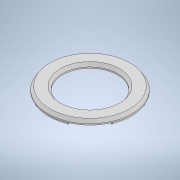
# Autodesk Inventor part: mirror_lock_v1
Saved by Autodesk Inventor 2020 (Build 240168000, 168)
## iProperties
Created: 2024-03-22
Part Number: mirror_lock_v1
Material: Типовые
Document SubType Name: Modeling
Designer: 4s
Density: 1 g/cm^3
Appearance: По умолчанию
Author: 4s
Autodesk Inventor part; units mm, degrees
ref_plane "YZ Plane" through (0, 0, 0) normal (1, 0, 0) x (0, 1, 0)
ref_plane "XZ Plane" through (0, 0, 0) normal (0, 1, 0) x (-1, 0, 0)
ref_plane "XY Plane" through (0, 0, 0) normal (0, 0, 1) x (1, 0, 0)
sketch "Эскиз1" plane through (0, 0, 0) normal (1, 0, 0) x (0, 1, 0)
  line L0 (0, 0) -> (13.9611, 0) construction
  line L1 (0, 26.35) -> (-10, 26.35) construction
  line L2 (-10, 26.35) -> (-10, -26.35) construction
  line L3 (-10, -26.35) -> (0, -26.35) construction
  line L4 (0, -26.35) -> (0, 26.35) construction
  line L5 (0, 0) -> (0, -22.0675) construction
  line L6 (2, 25) -> (0, 25) construction
  line L7 (0, 25) -> (0, -25) construction
  line L8 (0, -25) -> (2, -25) construction
  line L9 (2, -25) -> (2, 25) construction
  line L10 (5, -19) -> (5, -30.35)
  line L11 (-2, -11.433) -> (-2, -38.2242) construction
  line L12 (5, -19) -> (2, -19)
  line L13 (5, -30.35) -> (2, -30.35)
  line L14 (2, -30.35) -> (2, -19)
  dimension "d0" = 10
  dimension "d1" = 52.7
  dimension "d2" = 2
  dimension "d3" = 50
  dimension "d4" = 3
  dimension "d6" = 2
  dimension "d7" = 6
  dimension "d8" = 3
  dimension "d10" = 4
  constraints: 30 end point, 6 parallel, 4 horizontal, 3 perpendicular, 2 collinear, 2 vertical, 1 point on line, 2 other
  measures "d0" distance of L3.end L2.end
  measures "d1" distance of L3.end L1.start
  measures "d2" distance between parallel lines of L4 L9
  measures "d3" distance of L8.end L6.start
  measures "d4" distance between parallel lines of L9 L10
  measures "d6" distance between parallel lines of L4 L11
  measures "d7" distance between parallel lines of L8 L12
  measures "d8" distance of L10.end L13.end
  measures "d10" distance between parallel lines of L3 L13
revolve "Вращение1" add sketch "Эскиз1" angle 360 about axis through (0, 0, 0) along (0, 1, 0)
chamfer "Фаска1" distance 1.5 angle 55 1 edges at (0, 5, 19) measured on face at (0, 5, 19.5)
sketch "Эскиз2" plane through (0, 0, 0) normal (0, 0, 1) x (1, 0, 0)
  line L0 (-30.35, 5) -> (30.35, 5) construction
  line L1 (-30.35, 2) -> (30.35, 2) construction
  line L2 (-19, 2.8578) -> (19, 2.8578) construction
  line L3 (20.5, 5) -> (-20.5, 5) construction
  line L4 (-19, 2) -> (19, 2) construction
  line L5 (-19, 2.8578) -> (19, 2.8578) construction
  line L6 (0, 0) -> (25, 0) construction
  line L7 (25, 2) -> (25, -8.0068) construction
  line L8 (-30.35, 2) -> (30.35, 2) construction
  line L9 (26, 2) -> (26, -4.9803) construction
  line L10 (26.25, 1.5) -> (26.25, 1.5) construction
  line L11 (27, 1.5) -> (27, 0) construction
  line L12 (27, 0) -> (26.25, 0) construction
  line L13 (25.5, 0.75) -> (25.5, 0.75) construction
  line L14 (27, 0) -> (27, 0) construction
  line L15 (29, 2) -> (29, 2) construction
  line L16 (29, 2) -> (27, 2) construction
  line L17 (27, 2) -> (27, 2.25) construction
  arc A0 (26.25, 1.5) -> (25.5, 0.75) centre (26.25, 0.75) ccw
  arc A1 (25.5, 0.75) -> (26.25, 0) centre (26.25, 0.75) ccw
  arc A2 (27, 0) -> (29, 2) centre (27, 2) ccw
  line L18 (26.9571, 2) -> (29, 2)
  line L19 (26.25, 0) -> (27, 0)
  line L20 (-19, 2) -> (19, 2) projected
  line L21 (0, 2) -> (0, 5)
  line L22 (-30.35, 5) -> (30.35, 5) projected
  line L23 (26.25, 1.5) -> (26.9571, 2)
  point P0 (25.5, 0)
  dimension "d15" = 25
  dimension "d16" = 1
  dimension "d17" = 1.5
  dimension "d18" = 1.5
  dimension "d19" = 0.5
  dimension "d20" = 2
  dimension "d21" = 0.75
  dimension "d22" = 2
  constraints: 30 end point, 8 point on line, 7 tangent, 6 point on circle, 5 collinear, 4 parallel, 3 centre point, 3 horizontal, 3 perpendicular, 2 midpoint, 1 concentric, 1 vertical
  measures "d15" distance of L6.start L6.end
  measures "d16" distance between parallel lines of L7 L9
  measures "d17" distance of L11.end point (25.5, 0)
  measures "d18" distance of L11.start L11.end
  measures "d19" distance between parallel lines of L9 L13
  measures "d20" distance of L16.end L15.end
  measures "d21" radius of A0
  measures "d22" radius of A2
revolve "Вращение2" add sketch "Эскиз2" angle 45 mid plane about axis through (0, 2, 0) along (0, 1, 0)
pattern_circular "Круговой массив1" count 4 over 360 about axis through (0, 3.5, 0) along (0, -1, 0) of "Вращение2"
sketch "Эскиз3" plane through (0, 0, 0) normal (0, 0, 1) x (1, 0, 0)
  line L0 (-30.35, 5) -> (30.35, 5) construction
  line L1 (20.5, 5) -> (-20.5, 5) construction
  arc A0 (-29, 2) -> (-27, 0) centre (-27, 2) ccw construction
  line L2 (-29, 2) -> (-29, 5)
  line L3 (-29, 5) -> (-20.5, 5) construction
  line L4 (-29, 2) -> (-31.1266, 2)
  line L5 (-31.1266, 2) -> (-31.1266, 5.1774)
  line L6 (-31.1266, 5.1774) -> (-29, 5.1774)
  line L7 (-29, 5.1774) -> (-29, 2)
  line L8 (0, 0) -> (0, 5)
  constraints: 14 end point, 2 parallel, 2 perpendicular, 1 collinear, 1 horizontal, 1 midpoint, 1 point on line
revolve "Вращение3" cut sketch "Эскиз3" angle 360 about axis through (0, 0, 0) along (0, 1, 0)
chamfer "Фаска2" distance 1.5 angle 55 1 edges at (29, 5, 0) measured on face at (28.5, 5, 0)
